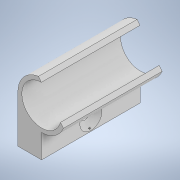
# Autodesk Inventor part: shadeHolderKetchenWindow
Saved by Autodesk Inventor 2022 (Build 260153070, 153G)
## iProperties
Created: 2021-02-12
Part Number: shadeHolderKetchenWindow
Material: Generic
Document SubType Name: Modeling
Designer: robst
Density: 1 g/cm^3
Appearance: Default
Author: robst
Autodesk Inventor part; units mm, degrees
ref_plane "YZ Plane" through (0, 0, 0) normal (1, 0, 0) x (0, 1, 0)
ref_plane "XZ Plane" through (0, 0, 0) normal (0, 1, 0) x (-1, 0, 0)
ref_plane "XY Plane" through (0, 0, 0) normal (0, 0, 1) x (1, 0, 0)
sketch "Sketch4" plane through (0, 0, 0) normal (0, 0, 1) x (1, 0, 0)
  arc A0 (-0.0698, 6.3496) -> (6.1152, -1.7109) centre (0, 0) ccw
  arc A1 (-0.9946, 7.5548) -> (7.04, -2.916) centre (0, 0) ccw
  line L0 (0, 0) -> (0, 7.9375) construction
  line L1 (-0.0698, 6.3496) -> (6.1152, -1.7109) construction
  line L2 (-0.0698, 6.3496) -> (-0.9946, 7.5548)
  line L3 (6.1152, -1.7109) -> (7.04, -2.916)
  circle A2 centre (0, 0) radius 6.35
  dimension "d10" = 12.7
  dimension "d11" = 1.27
  dimension "d12" = 37.5
  dimension "d13" = 10.16
  constraints: 8 end point, 4 point on circle, 3 centre point, 3 coincident, 1 collinear, 1 concentric, 1 point on line, 1 vertical
  measures "d10" diameter of A0
  measures "d11" radial gap between concentric circles of A1 A0
  measures "d12" angle of L1 L0
  measures "d13" distance of L1.start L1.end
extrude "Extrusion3" add sketch "Sketch4" along normal mid plane 31.75 contours A0 L3 A1 L2
sketch "Sketch5" plane through (0, 0, 0) normal (0, 0, 1) x (1, 0, 0)
  arc A0 (-0.9946, 7.5548) -> (7.04, -2.916) centre (0, 0) ccw projected
  line L0 (-7.62, 0) -> (-7.62, -15.24)
  line L1 (-7.62, -15.24) -> (0, -15.24)
  line L2 (0, -15.24) -> (0, -7.62)
  circle A1 centre (0, 0) radius 7.9375
  dimension "d16" = 7.62
  constraints: 6 end point, 2 perpendicular, 2 point on circle, 1 centre point, 1 coincident, 1 tangent, 1 vertical
  measures "d16" distance from line of L2.end L1
extrude "Extrusion4" add sketch "Sketch5" along normal mid plane 31.75 contours A0 L2 A1 L0 | A1 L2 L1 L0 picked at (-7.3048, -2.4081)
sketch "Sketch6" plane through (0, -15.24, 15.875) normal (1, 0, 0) x (0, 0, -1)
  line L0 (0, 7.62) -> (31.75, 7.62) projected
  line L1 (31.75, 7.62) -> (31.75, 0) projected
  line L2 (0, 0) -> (31.75, 0) projected
  line L3 (0, 0) -> (0, 7.62) projected
  line L4 (0, 7.62) -> (31.75, 0) construction
  line L5 (31.75, 7.62) -> (0, 0) construction
  point P0 (15.875, 15.24)
  point P1 (15.875, 3.81)
  constraints: 4 end point, 1 midpoint
hole "Hole1" at (0, -11.43, 0) direction (-1, 0, 0) diameter 3.5052 end through all countersink diameter 7.112 countersink angle 82
sketch "Sketch10" plane through (-7.62, -15.24, 15.875) normal (0, -1, 0) x (1, 0, 0)
  line L0 (0, -31.75) -> (0, 0) projected
  line L1 (7.62, -31.75) -> (0, -31.75) projected
  line L2 (7.62, 0) -> (7.62, -31.75) projected
  line L3 (0, 0) -> (7.62, 0) projected
  line L4 (3.81, -31.75) -> (3.81, 0) construction
  line L5 (3.175, -26.67) -> (3.175, -27.1084)
  line L6 (3.175, -27.1084) -> (1.9935, -28.0367)
  line L7 (1.9935, -28.0367) -> (2.1602, -28.1849)
  line L8 (2.1602, -28.1849) -> (3.175, -28.1849)
  line L9 (3.175, -28.1849) -> (3.175, -28.5225)
  line L10 (3.175, -28.5225) -> (0.635, -28.5225)
  line L11 (0.635, -28.5225) -> (0.635, -28.1849)
  line L12 (0.635, -28.1849) -> (1.8021, -28.1849)
  line L13 (1.8021, -28.1849) -> (0.635, -27.1434)
  line L14 (0.635, -27.1434) -> (0.635, -26.7318)
  line L15 (0.635, -26.7318) -> (1.7691, -27.7836)
  line L16 (1.7691, -27.7836) -> (3.175, -26.67)
  spline S0 degree 2 poles (3.2182, -25.6655) (3.2182, -26.1225) (2.7057, -26.6247) (2.2323, -26.6247) knots 0 0 0 1 2 2 2
  spline S1 degree 2 poles (2.2323, -26.6247) (1.7671, -26.6247) (1.2155, -26.1369) (1.2155, -25.7437) knots 0 0 0 1 2 2 2
  spline S2 degree 2 poles (1.2155, -25.7437) (1.2155, -25.5667) (1.3184, -25.293) (1.4275, -25.1921) knots 0 0 0 1 2 2 2
  spline S3 degree 2 poles (1.4275, -25.1921) (1.5366, -25.0892) (1.8515, -24.9801) (2.08, -24.9801) knots 0 0 0 1 2 2 2
  line L17 (2.08, -24.9801) -> (2.2549, -24.9801)
  line L18 (2.2549, -24.9801) -> (2.2549, -26.2995)
  spline S4 degree 2 poles (2.2549, -26.2995) (2.5863, -26.2995) (2.9383, -25.966) (2.9383, -25.6696) knots 0 0 0 1 2 2 2
  spline S5 degree 2 poles (2.9383, -25.6696) (2.9383, -25.5647) (2.8909, -25.3609) (2.8539, -25.2786) knots 0 0 0 1 2 2 2
  spline S6 degree 2 poles (2.8539, -25.2786) (2.8127, -25.1921) (2.7407, -25.0727) (2.7078, -25.0336) knots 0 0 0 1 2 2 2
  line L19 (2.7078, -25.0336) -> (2.7078, -25.0151)
  line L20 (2.7078, -25.0151) -> (3.0577, -25.0151)
  spline S7 degree 2 poles (3.0577, -25.0151) (3.0803, -25.0707) (3.1462, -25.2394) (3.1647, -25.3053) knots 0 0 0 1 2 2 2
  spline S8 degree 2 poles (3.1647, -25.3053) (3.1915, -25.3979) (3.2182, -25.5503) (3.2182, -25.6655) knots 0 0 0 1 2 2 2
  spline S9 degree 2 poles (2.01, -25.293) (1.8803, -25.2971) (1.6909, -25.3506) (1.6271, -25.4021) knots 0 0 0 1 2 2 2
  spline S10 degree 2 poles (1.6271, -25.4021) (1.5551, -25.4576) (1.4789, -25.6326) (1.4789, -25.7623) knots 0 0 0 1 2 2 2
  spline S11 degree 2 poles (1.4789, -25.7623) (1.4789, -25.8899) (1.5551, -26.069) (1.6292, -26.1431) knots 0 0 0 1 2 2 2
  spline S12 degree 2 poles (1.6292, -26.1431) (1.7053, -26.2151) (1.8885, -26.2892) (2.01, -26.2995) knots 0 0 0 1 2 2 2
  line L21 (2.01, -26.2995) -> (2.01, -25.293)
  spline S13 degree 2 poles (3.2121, -24.0785) (3.2121, -24.34) (2.9136, -24.6343) (2.5904, -24.6343) knots 0 0 0 1 2 2 2
  line L22 (2.5904, -24.6343) -> (1.5345, -24.6343)
  line L23 (1.5345, -24.6343) -> (1.5345, -24.8504)
  line L24 (1.5345, -24.8504) -> (1.269, -24.8504)
  line L25 (1.269, -24.8504) -> (1.269, -24.6343)
  line L26 (1.269, -24.6343) -> (0.7215, -24.6343)
  line L27 (0.7215, -24.6343) -> (0.7215, -24.3132)
  line L28 (0.7215, -24.3132) -> (1.269, -24.3132)
  line L29 (1.269, -24.3132) -> (1.269, -23.7224)
  line L30 (1.269, -23.7224) -> (1.5345, -23.7224)
  line L31 (1.5345, -23.7224) -> (1.5345, -24.3132)
  line L32 (1.5345, -24.3132) -> (2.4422, -24.3132)
  spline S14 degree 2 poles (2.4422, -24.3132) (2.5863, -24.3132) (2.7448, -24.3029) (2.8127, -24.2679) knots 0 0 0 1 2 2 2
  spline S15 degree 2 poles (2.8127, -24.2679) (2.8724, -24.2391) (2.9321, -24.1094) (2.9321, -23.9983) knots 0 0 0 1 2 2 2
  spline S16 degree 2 poles (2.9321, -23.9983) (2.9321, -23.92) (2.8848, -23.7739) (2.8704, -23.741) knots 0 0 0 1 2 2 2
  line L33 (2.8704, -23.741) -> (2.8704, -23.7224)
  line L34 (2.8704, -23.7224) -> (3.1585, -23.7224)
  spline S17 degree 2 poles (3.1585, -23.7224) (3.1832, -23.813) (3.2121, -23.9983) (3.2121, -24.0785) knots 0 0 0 1 2 2 2
  spline S18 degree 2 poles (3.2182, -22.7283) (3.2182, -22.9259) (3.0968, -23.2531) (2.9733, -23.3705) knots 0 0 0 1 2 2 2
  spline S19 degree 2 poles (2.9733, -23.3705) (2.8518, -23.4878) (2.4772, -23.6175) (2.2261, -23.6175) knots 0 0 0 1 2 2 2
  spline S20 degree 2 poles (2.2261, -23.6175) (1.975, -23.6175) (1.6086, -23.4837) (1.4851, -23.3705) knots 0 0 0 1 2 2 2
  spline S21 degree 2 poles (1.4851, -23.3705) (1.3595, -23.2573) (1.2257, -22.9218) (1.2257, -22.7283) knots 0 0 0 1 2 2 2
  spline S22 degree 2 poles (1.2257, -22.7283) (1.2257, -22.5718) (1.3143, -22.2795) (1.3719, -22.1663) knots 0 0 0 1 2 2 2
  line L35 (1.3719, -22.1663) -> (1.7321, -22.1663)
  line L36 (1.7321, -22.1663) -> (1.7321, -22.1849)
  spline S23 degree 2 poles (1.7321, -22.1849) (1.7033, -22.2199) (1.6292, -22.3269) (1.5901, -22.403) knots 0 0 0 1 2 2 2
  spline S24 degree 2 poles (1.5901, -22.403) (1.5571, -22.471) (1.5057, -22.6521) (1.5057, -22.7344) knots 0 0 0 1 2 2 2
  spline S25 degree 2 poles (1.5057, -22.7344) (1.5057, -22.9835) (1.8824, -23.2861) (2.2261, -23.2861) knots 0 0 0 1 2 2 2
  spline S26 degree 2 poles (2.2261, -23.2861) (2.5616, -23.2861) (2.9383, -22.9938) (2.9383, -22.7344) knots 0 0 0 1 2 2 2
  spline S27 degree 2 poles (2.9383, -22.7344) (2.9383, -22.578) (2.8086, -22.294) (2.7078, -22.1849) knots 0 0 0 1 2 2 2
  line L37 (2.7078, -22.1849) -> (2.7078, -22.1663)
  line L38 (2.7078, -22.1663) -> (3.068, -22.1663)
  spline S28 degree 2 poles (3.068, -22.1663) (3.0906, -22.2137) (3.1544, -22.3578) (3.1688, -22.4154) knots 0 0 0 1 2 2 2
  spline S29 degree 2 poles (3.1688, -22.4154) (3.1935, -22.4977) (3.2182, -22.6274) (3.2182, -22.7283) knots 0 0 0 1 2 2 2
  line L39 (3.175, -20.3776) -> (3.175, -20.6987)
  line L40 (3.175, -20.6987) -> (2.0882, -20.6987)
  spline S30 degree 2 poles (2.0882, -20.6987) (1.9565, -20.6987) (1.73, -20.7234) (1.6621, -20.7605) knots 0 0 0 1 2 2 2
  spline S31 degree 2 poles (1.6621, -20.7605) (1.5901, -20.7996) (1.5201, -20.9396) (1.5201, -21.0589) knots 0 0 0 1 2 2 2
  spline S32 degree 2 poles (1.5201, -21.0589) (1.5201, -21.1783) (1.6477, -21.4315) (1.7506, -21.553) knots 0 0 0 1 2 2 2
  line L41 (1.7506, -21.553) -> (3.175, -21.553)
  line L42 (3.175, -21.553) -> (3.175, -21.8741)
  line L43 (3.175, -21.8741) -> (0.5218, -21.8741)
  line L44 (0.5218, -21.8741) -> (0.5218, -21.553)
  line L45 (0.5218, -21.553) -> (1.481, -21.553)
  spline S33 degree 2 poles (1.481, -21.553) (1.3513, -21.4089) (1.2155, -21.131) (1.2155, -20.9746) knots 0 0 0 1 2 2 2
  spline S34 degree 2 poles (1.2155, -20.9746) (1.2155, -20.6946) (1.586, -20.3776) (1.9379, -20.3776) knots 0 0 0 1 2 2 2
  line L46 (1.9379, -20.3776) -> (3.175, -20.3776)
  spline S35 degree 2 poles (3.2182, -19.0994) (3.2182, -19.5564) (2.7057, -20.0586) (2.2323, -20.0586) knots 0 0 0 1 2 2 2
  spline S36 degree 2 poles (2.2323, -20.0586) (1.7671, -20.0586) (1.2155, -19.5708) (1.2155, -19.1776) knots 0 0 0 1 2 2 2
  spline S37 degree 2 poles (1.2155, -19.1776) (1.2155, -19.0006) (1.3184, -18.7268) (1.4275, -18.626) knots 0 0 0 1 2 2 2
  spline S38 degree 2 poles (1.4275, -18.626) (1.5366, -18.5231) (1.8515, -18.414) (2.08, -18.414) knots 0 0 0 1 2 2 2
  line L47 (2.08, -18.414) -> (2.2549, -18.414)
  line L48 (2.2549, -18.414) -> (2.2549, -19.7334)
  spline S39 degree 2 poles (2.2549, -19.7334) (2.5863, -19.7334) (2.9383, -19.3999) (2.9383, -19.1035) knots 0 0 0 1 2 2 2
  spline S40 degree 2 poles (2.9383, -19.1035) (2.9383, -18.9985) (2.8909, -18.7948) (2.8539, -18.7124) knots 0 0 0 1 2 2 2
  spline S41 degree 2 poles (2.8539, -18.7124) (2.8127, -18.626) (2.7407, -18.5066) (2.7078, -18.4675) knots 0 0 0 1 2 2 2
  line L49 (2.7078, -18.4675) -> (2.7078, -18.449)
  line L50 (2.7078, -18.449) -> (3.0577, -18.449)
  spline S42 degree 2 poles (3.0577, -18.449) (3.0803, -18.5045) (3.1462, -18.6733) (3.1647, -18.7392) knots 0 0 0 1 2 2 2
  spline S43 degree 2 poles (3.1647, -18.7392) (3.1915, -18.8318) (3.2182, -18.9841) (3.2182, -19.0994) knots 0 0 0 1 2 2 2
  spline S44 degree 2 poles (2.01, -18.7268) (1.8803, -18.731) (1.6909, -18.7845) (1.6271, -18.8359) knots 0 0 0 1 2 2 2
  spline S45 degree 2 poles (1.6271, -18.8359) (1.5551, -18.8915) (1.4789, -19.0665) (1.4789, -19.1961) knots 0 0 0 1 2 2 2
  spline S46 degree 2 poles (1.4789, -19.1961) (1.4789, -19.3238) (1.5551, -19.5028) (1.6292, -19.5769) knots 0 0 0 1 2 2 2
  spline S47 degree 2 poles (1.6292, -19.5769) (1.7053, -19.649) (1.8885, -19.7231) (2.01, -19.7334) knots 0 0 0 1 2 2 2
  line L51 (2.01, -19.7334) -> (2.01, -18.7268)
  line L52 (3.175, -16.5923) -> (3.175, -16.9134)
  line L53 (3.175, -16.9134) -> (2.0882, -16.9134)
  spline S48 degree 2 poles (2.0882, -16.9134) (1.9565, -16.9134) (1.73, -16.9381) (1.6621, -16.9752) knots 0 0 0 1 2 2 2
  spline S49 degree 2 poles (1.6621, -16.9752) (1.5901, -17.0143) (1.5201, -17.1543) (1.5201, -17.2736) knots 0 0 0 1 2 2 2
  spline S50 degree 2 poles (1.5201, -17.2736) (1.5201, -17.393) (1.6477, -17.6462) (1.7506, -17.7677) knots 0 0 0 1 2 2 2
  line L54 (1.7506, -17.7677) -> (3.175, -17.7677)
  line L55 (3.175, -17.7677) -> (3.175, -18.0888)
  line L56 (3.175, -18.0888) -> (1.269, -18.0888)
  line L57 (1.269, -18.0888) -> (1.269, -17.7677)
  line L58 (1.269, -17.7677) -> (1.481, -17.7677)
  spline S51 degree 2 poles (1.481, -17.7677) (1.3513, -17.6236) (1.2155, -17.3457) (1.2155, -17.1893) knots 0 0 0 1 2 2 2
  spline S52 degree 2 poles (1.2155, -17.1893) (1.2155, -16.9093) (1.586, -16.5923) (1.9379, -16.5923) knots 0 0 0 1 2 2 2
  line L59 (1.9379, -16.5923) -> (3.175, -16.5923)
  line L60 (0.635, -12.1792) -> (3.175, -12.8173)
  line L61 (3.175, -12.8173) -> (3.175, -13.1961)
  line L62 (3.175, -13.1961) -> (1.0673, -13.7127)
  line L63 (1.0673, -13.7127) -> (3.175, -14.2149)
  line L64 (3.175, -14.2149) -> (3.175, -14.5896)
  line L65 (3.175, -14.5896) -> (0.635, -15.2379)
  line L66 (0.635, -15.2379) -> (0.635, -14.8901)
  line L67 (0.635, -14.8901) -> (2.7407, -14.3796)
  line L68 (2.7407, -14.3796) -> (0.635, -13.8733)
  line L69 (0.635, -13.8733) -> (0.635, -13.5295)
  line L70 (0.635, -13.5295) -> (2.7654, -13.019)
  line L71 (2.7654, -13.019) -> (0.635, -12.5106)
  line L72 (0.635, -12.5106) -> (0.635, -12.1792)
  line L73 (3.175, -11.5741) -> (3.175, -11.8952)
  line L74 (3.175, -11.8952) -> (1.269, -11.8952)
  line L75 (1.269, -11.8952) -> (1.269, -11.5741)
  line L76 (1.269, -11.5741) -> (3.175, -11.5741)
  line L77 (0.952, -11.5514) -> (0.952, -11.9158)
  line L78 (0.952, -11.9158) -> (0.6185, -11.9158)
  line L79 (0.6185, -11.9158) -> (0.6185, -11.5514)
  line L80 (0.6185, -11.5514) -> (0.952, -11.5514)
  line L81 (3.175, -9.6063) -> (3.175, -9.9274)
  line L82 (3.175, -9.9274) -> (2.0882, -9.9274)
  spline S53 degree 2 poles (2.0882, -9.9274) (1.9565, -9.9274) (1.73, -9.9521) (1.6621, -9.9892) knots 0 0 0 1 2 2 2
  spline S54 degree 2 poles (1.6621, -9.9892) (1.5901, -10.0283) (1.5201, -10.1682) (1.5201, -10.2876) knots 0 0 0 1 2 2 2
  spline S55 degree 2 poles (1.5201, -10.2876) (1.5201, -10.407) (1.6477, -10.6602) (1.7506, -10.7816) knots 0 0 0 1 2 2 2
  line L83 (1.7506, -10.7816) -> (3.175, -10.7816)
  line L84 (3.175, -10.7816) -> (3.175, -11.1027)
  line L85 (3.175, -11.1027) -> (1.269, -11.1027)
  line L86 (1.269, -11.1027) -> (1.269, -10.7816)
  line L87 (1.269, -10.7816) -> (1.481, -10.7816)
  spline S56 degree 2 poles (1.481, -10.7816) (1.3513, -10.6375) (1.2155, -10.3597) (1.2155, -10.2032) knots 0 0 0 1 2 2 2
  spline S57 degree 2 poles (1.2155, -10.2032) (1.2155, -9.9233) (1.586, -9.6063) (1.9379, -9.6063) knots 0 0 0 1 2 2 2
  line L88 (1.9379, -9.6063) -> (3.175, -9.6063)
  line L89 (3.175, -7.69) -> (3.175, -8.0111)
  line L90 (3.175, -8.0111) -> (2.9815, -8.0111)
  spline S58 degree 2 poles (2.9815, -8.0111) (3.0433, -8.0852) (3.1256, -8.1943) (3.1606, -8.2684) knots 0 0 0 1 2 2 2
  spline S59 degree 2 poles (3.1606, -8.2684) (3.1935, -8.3363) (3.2285, -8.4824) (3.2285, -8.5792) knots 0 0 0 1 2 2 2
  spline S60 degree 2 poles (3.2285, -8.5792) (3.2285, -8.7356) (3.0988, -8.9991) (2.9733, -9.0917) knots 0 0 0 1 2 2 2
  spline S61 degree 2 poles (2.9733, -9.0917) (2.8477, -9.1843) (2.4772, -9.2873) (2.2364, -9.2873) knots 0 0 0 1 2 2 2
  spline S62 degree 2 poles (2.2364, -9.2873) (1.9853, -9.2873) (1.6189, -9.1576) (1.481, -9.0444) knots 0 0 0 1 2 2 2
  spline S63 degree 2 poles (1.481, -9.0444) (1.3575, -8.9394) (1.2155, -8.6451) (1.2155, -8.4824) knots 0 0 0 1 2 2 2
  spline S64 degree 2 poles (1.2155, -8.4824) (1.2155, -8.3404) (1.2793, -8.1284) (1.3451, -8.0111) knots 0 0 0 1 2 2 2
  line L91 (1.3451, -8.0111) -> (0.5218, -8.0111)
  line L92 (0.5218, -8.0111) -> (0.5218, -7.69)
  line L93 (0.5218, -7.69) -> (3.175, -7.69)
  line L94 (2.7119, -8.0111) -> (1.6107, -8.0111)
  spline S65 degree 2 poles (1.6107, -8.0111) (1.553, -8.1305) (1.5098, -8.3198) (1.5098, -8.4289) knots 0 0 0 1 2 2 2
  spline S66 degree 2 poles (1.5098, -8.4289) (1.5098, -8.6759) (1.8803, -8.9559) (2.2302, -8.9559) knots 0 0 0 1 2 2 2
  spline S67 degree 2 poles (2.2302, -8.9559) (2.5678, -8.9559) (2.9239, -8.7418) (2.9239, -8.5051) knots 0 0 0 1 2 2 2
  spline S68 degree 2 poles (2.9239, -8.5051) (2.9239, -8.3795) (2.8086, -8.1243) (2.7119, -8.0111) knots 0 0 0 1 2 2 2
  spline S69 degree 2 poles (2.222, -5.6584) (2.7036, -5.6584) (3.2285, -6.1215) (3.2285, -6.5085) knots 0 0 0 1 2 2 2
  spline S70 degree 2 poles (3.2285, -6.5085) (3.2285, -6.9058) (2.6872, -7.3606) (2.222, -7.3606) knots 0 0 0 1 2 2 2
  spline S71 degree 2 poles (2.222, -7.3606) (1.7444, -7.3606) (1.2155, -6.8913) (1.2155, -6.5085) knots 0 0 0 1 2 2 2
  spline S72 degree 2 poles (1.2155, -6.5085) (1.2155, -6.1215) (1.7424, -5.6584) (2.222, -5.6584) knots 0 0 0 1 2 2 2
  spline S73 degree 2 poles (2.222, -5.9898) (1.8515, -5.9898) (1.4913, -6.2594) (1.4913, -6.5085) knots 0 0 0 1 2 2 2
  spline S74 degree 2 poles (1.4913, -6.5085) (1.4913, -6.7576) (1.8515, -7.0293) (2.222, -7.0293) knots 0 0 0 1 2 2 2
  spline S75 degree 2 poles (2.222, -7.0293) (2.5822, -7.0293) (2.9527, -6.7576) (2.9527, -6.5085) knots 0 0 0 1 2 2 2
  spline S76 degree 2 poles (2.9527, -6.5085) (2.9527, -6.2615) (2.5884, -5.9898) (2.222, -5.9898) knots 0 0 0 1 2 2 2
  line L95 (1.269, -3.0196) -> (3.175, -3.5033)
  line L96 (3.175, -3.5033) -> (3.175, -3.7997)
  line L97 (3.175, -3.7997) -> (1.7053, -4.2649)
  line L98 (1.7053, -4.2649) -> (3.175, -4.728)
  line L99 (3.175, -4.728) -> (3.175, -5.0224)
  line L100 (3.175, -5.0224) -> (1.269, -5.5102)
  line L101 (1.269, -5.5102) -> (1.269, -5.1767)
  line L102 (1.269, -5.1767) -> (2.7448, -4.8392)
  line L103 (2.7448, -4.8392) -> (1.269, -4.3884)
  line L104 (1.269, -4.3884) -> (1.269, -4.1229)
  line L105 (1.269, -4.1229) -> (2.7448, -3.6597)
  line L106 (2.7448, -3.6597) -> (1.269, -3.3428)
  line L107 (1.269, -3.3428) -> (1.269, -3.0196)
  spline S77 degree 2 poles (5.5416, -16.9711) (5.7063, -16.9711) (6.0027, -17.0884) (6.1056, -17.1934) knots 0 0 0 1 2 2 2
  spline S78 degree 2 poles (6.1056, -17.1934) (6.2353, -17.3251) (6.3691, -17.6812) (6.3691, -17.9529) knots 0 0 0 1 2 2 2
  line L108 (6.3691, -17.9529) -> (6.3691, -18.239)
  line L109 (6.3691, -18.239) -> (7.3159, -18.239)
  line L110 (7.3159, -18.239) -> (7.3159, -18.5766)
  line L111 (7.3159, -18.5766) -> (4.7759, -18.5766)
  line L112 (4.7759, -18.5766) -> (4.7759, -17.9385)
  spline S79 degree 2 poles (4.7759, -17.9385) (4.7759, -17.7121) (4.85, -17.3951) (4.9344, -17.2736) knots 0 0 0 1 2 2 2
  spline S80 degree 2 poles (4.9344, -17.2736) (5.0312, -17.1316) (5.3296, -16.9711) (5.5416, -16.9711) knots 0 0 0 1 2 2 2
  spline S81 degree 2 poles (5.5519, -17.323) (5.4202, -17.323) (5.2267, -17.4136) (5.165, -17.5062) knots 0 0 0 1 2 2 2
  spline S82 degree 2 poles (5.165, -17.5062) (5.1114, -17.5865) (5.0682, -17.8006) (5.0682, -17.9591) knots 0 0 0 1 2 2 2
  line L113 (5.0682, -17.9591) -> (5.0682, -18.239)
  line L114 (5.0682, -18.239) -> (6.0809, -18.239)
  line L115 (6.0809, -18.239) -> (6.0809, -18.0085)
  spline S83 degree 2 poles (6.0809, -18.0085) (6.0809, -17.8026) (6.0151, -17.5495) (5.9286, -17.4671) knots 0 0 0 1 2 2 2
  spline S84 degree 2 poles (5.9286, -17.4671) (5.8525, -17.391) (5.6734, -17.323) (5.5519, -17.323) knots 0 0 0 1 2 2 2
  line L116 (4.7759, -14.8077) -> (7.3159, -15.6825)
  line L117 (7.3159, -15.6825) -> (7.3159, -16.0469)
  line L118 (7.3159, -16.0469) -> (4.7759, -16.9217)
  line L119 (4.7759, -16.9217) -> (4.7759, -16.5594)
  line L120 (4.7759, -16.5594) -> (6.8857, -15.8554)
  line L121 (6.8857, -15.8554) -> (4.7759, -15.1515)
  line L122 (4.7759, -15.1515) -> (4.7759, -14.8077)
  spline S85 degree 2 poles (6.5091, -13.0684) (6.6923, -13.0684) (7.0051, -13.1858) (7.1204, -13.2928) knots 0 0 0 1 2 2 2
  spline S86 degree 2 poles (7.1204, -13.2928) (7.2357, -13.3998) (7.3695, -13.7189) (7.3695, -13.9165) knots 0 0 0 1 2 2 2
  spline S87 degree 2 poles (7.3695, -13.9165) (7.3695, -14.0976) (7.2892, -14.4517) (7.2254, -14.5813) knots 0 0 0 1 2 2 2
  line L123 (7.2254, -14.5813) -> (6.8652, -14.5813)
  line L124 (6.8652, -14.5813) -> (6.8652, -14.5566)
  spline S88 degree 2 poles (6.8652, -14.5566) (6.894, -14.5175) (6.9681, -14.3714) (7.001, -14.2829) knots 0 0 0 1 2 2 2
  spline S89 degree 2 poles (7.001, -14.2829) (7.036, -14.182) (7.0751, -14.0153) (7.0751, -13.9103) knots 0 0 0 1 2 2 2
  spline S90 degree 2 poles (7.0751, -13.9103) (7.0751, -13.8074) (7.001, -13.6139) (6.9207, -13.5439) knots 0 0 0 1 2 2 2
  spline S91 degree 2 poles (6.9207, -13.5439) (6.8446, -13.4801) (6.6429, -13.4142) (6.507, -13.4142) knots 0 0 0 1 2 2 2
  spline S92 degree 2 poles (6.507, -13.4142) (6.3712, -13.4142) (6.1983, -13.4883) (6.1406, -13.5583) knots 0 0 0 1 2 2 2
  spline S93 degree 2 poles (6.1406, -13.5583) (6.0768, -13.6304) (6.0233, -13.8444) (6.0233, -13.9741) knots 0 0 0 1 2 2 2
  spline S94 degree 2 poles (6.0233, -13.9741) (6.0233, -14.1141) (6.0665, -14.392) (6.085, -14.4764) knots 0 0 0 1 2 2 2
  line L125 (6.085, -14.4764) -> (4.7759, -14.4764)
  line L126 (4.7759, -14.4764) -> (4.7759, -13.0829)
  line L127 (4.7759, -13.0829) -> (5.0744, -13.0829)
  line L128 (5.0744, -13.0829) -> (5.0744, -14.1491)
  line L129 (5.0744, -14.1491) -> (5.7516, -14.1491)
  spline S95 degree 2 poles (5.7516, -14.1491) (5.7434, -14.0873) (5.7372, -13.9679) (5.7372, -13.9185) knots 0 0 0 1 2 2 2
  spline S96 degree 2 poles (5.7372, -13.9185) (5.7372, -13.723) (5.801, -13.4534) (5.8957, -13.3299) knots 0 0 0 1 2 2 2
  spline S97 degree 2 poles (5.8957, -13.3299) (5.9904, -13.2043) (6.2785, -13.0684) (6.5091, -13.0684) knots 0 0 0 1 2 2 2
  point P0 (7.62, -15.875)
  constraints: 2 end point, 2 midpoint, 1 vertical
extrude "Text" cut sketch "Sketch10" against normal blind 0.762 contours L5 L6 L7 L8 L9 L10 L11 L12 L13 L14 L15 L16 | S0 S1 S2 S3 L17 L18 S4 S5 S6 L19 L20 S7 S8 | S13 L22 L23 L24 L25 L26 L27 L28 L29 L30 L31 L32 S14 S15 S16 L33 L34 S17 | S18 S19 S20 S21 S22 L35 L36 S23 S24 S25 S26 S27 L37 L38 S28 S29 | L39 L40 S30 S31 S32 L41 L42 L43 L44 L45 S33 S34 L46 | S35 S36 S37 S38 L47 L48 S39 S40 S41 L49 L50 S42 S43 | L52 L53 S48 S49 S50 L54 L55 L56 L57 L58 S51 S52 L59 | L60 L61 L62 L63 L64 L65 L66 L67 L68 L69 L70 L71 L72 | L73 L74 L75 L76 | L77 L78 L79 L80 | L81 L82 S53 S54 S55 L83 L84 L85 L86 L87 S56 S57 L88 | L89 L90 S58 S59 S60 S61 S62 S63 S64 L91 L92 L93 | S69 S70 S71 S72 | L95 L96 L97 L98 L99 L100 L101 L102 L103 L104 L105 L106 L107 | S77 S78 L108 L109 L110 L111 L112 S79 S80 | L116 L117 L118 L119 L120 L121 L122 | S85 S86 S87 L123 L124 S88 S89 S90 S91 S92 S93 S94 L125 L126 L127 L128 L129 S95 S96 S97
equation "\"d10\" = shadeDiameter"
equation "\"d11\" = shadeHolderWallThickness"
equation "\"d13\" = openingForShade"
equation "\"d14\" = partWidth"
equation "\"d16\" = flatBelowShade"
equation "\"d17\" = partWidth"
equation "\"d28\" = textDepth"
equation "\"shadeDiameter\" = 12.7"
equation "\"partWidth\" = 31.75"
equation "\"backThickness\" = 1.905"
equation "\"backHeight\" = 25.4"
equation "\"cutTiltAngle\" = 52.5deg"
equation "\"flatBelowShade\" = 7.62"
equation "\"shadeHolderWallThickness\" = 1.27"
equation "\"openingForShade\" = 10.16"
equation "\"textDepth\" = 0.762"
body "Solid2"
